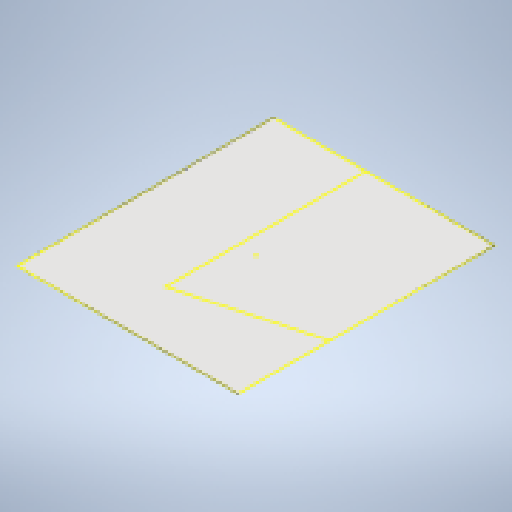
# Autodesk Inventor part: Top
Saved by Autodesk Inventor 2025.2 (Build 292293000, 293)
## iProperties
Created: 2025-05-26
Part Number: Top
Material: Generic
Document SubType Name: Sheet Metal
Designer: abdal
Density: 1 g/cm^3
Sheet Metal Rule: Default_mm
Appearance: Default
Author: abdal
Autodesk Inventor part; units mm, degrees
ref_plane "YZ Plane" through (0, 0, 0) normal (1, 0, 0) x (0, 1, 0)
ref_plane "XZ Plane" through (0, 0, 0) normal (0, 1, 0) x (-1, 0, 0)
ref_plane "XY Plane" through (0, 0, 0) normal (0, 0, 1) x (1, 0, 0)
sketch "Sketch1" plane through (0, 0, 0) normal (0, 1, 0) x (-1, 0, 0)
  line L0 (659.75, 765) -> (-659.75, 765)
  line L1 (-659.75, 765) -> (-659.75, -765)
  line L2 (-659.75, -765) -> (659.75, -765)
  line L3 (659.75, -765) -> (659.75, 765)
  line L4 (659.75, 765) -> (-659.75, -765) construction
  line L5 (-659.75, 765) -> (659.75, -765) construction
  point P0 (0, 0)
  dimension "d0" = 1319.5
  dimension "d1" = 1530
  measures "d0" distance of L1.end L2.end
  measures "d1" distance of L2.end L0.start
extrude "Plate1" add sketch "Sketch1" along normal blind 2
sketch "Sketch2" plane through (0, 2, 0) normal (0, 1, 0) x (1, 0, 0)
  line L0 (-108.25, -435) -> (-108.25, 765) projected
  line L1 (-108.25, -430.2912) -> (661.75, -217.4503) projected
  line L2 (659.75, -765) -> (-659.75, -765) projected
  line L3 (659.75, 765) -> (659.75, -765) projected
  line L4 (-659.75, 765) -> (659.75, 765) projected
  line L5 (-659.75, -765) -> (-659.75, 765) projected
  point P0 (0, 0)
  point P1 (659.75, -218.0031)
extrude "Extrusion1" cut sketch "Sketch2" against normal through all contours L0 L4 L3 L1
equation "\"d2\" = Thickness"
equation "\"BendRadius\" = Thickness"
equation "\"BendReliefWidth\" = Thickness"
equation "\"BendReliefDepth\" = 0.5 * Thickness"
equation "\"CornerReliefSize\" = 4 * Thickness"
equation "\"MinimumRemnant\" = 2 * Thickness"
equation "\"TransitionRadius\" = BendRadius"
equation "\"JacobiRadiusSize\" = BendRadius"
equation "\"GapSize\" = Thickness"
equation "\"Thickness\" = 2"
body "Solid1"
